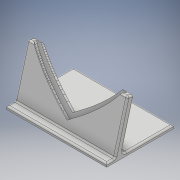
# Autodesk Inventor part: Supporto4
Saved by Autodesk Inventor 2018 (Build 220112000, 112)
## iProperties
Created: 2020-01-19
Part Number: Supporto4
Material: Generic
Document SubType Name: Modeling
Designer: Lorenzo Spadaro
Density: 1 g/cm^3
Appearance: Default
Author: Lorenzo Spadaro
Autodesk Inventor part; units mm, degrees
ref_plane "YZ Plane" through (0, 0, 0) normal (1, 0, 0) x (0, 1, 0)
ref_plane "XZ Plane" through (0, 0, 0) normal (0, 1, 0) x (-1, 0, 0)
ref_plane "XY Plane" through (0, 0, 0) normal (0, 0, 1) x (1, 0, 0)
sketch "Sketch1" plane through (0, 0, 0) normal (0, 0, 1) x (1, 0, 0)
  line L0 (-30, -20) -> (30, -20)
  line L1 (30, -20) -> (30, 20)
  line L2 (30, 20) -> (-30, 20)
  line L3 (-30, 20) -> (-30, -20)
  line L4 (-30, -20) -> (30, 20) construction
  line L5 (30, -20) -> (-30, 20) construction
  point P0 (0, 0)
  dimension "d0" = 60
  dimension "d1" = 40
  constraints: 12 end point, 2 midpoint, 2 parallel, 1 horizontal, 1 perpendicular
  measures "d0" distance of L2.end L1.end
  measures "d1" distance of L1.end L0.end
extrude "Extrusion1" add sketch "Sketch1" along normal blind 3
sketch "Sketch2" plane through (-30, -20, 0) normal (-1, 0, 0) x (0, 0, 1)
  line L0 (0, 0) -> (0, 40) projected
  line L1 (3, 40) -> (0, 40)
  line L2 (0, 40) -> (0, 0)
  line L3 (0, 0) -> (3, 0)
  line L4 (0, 40) -> (0, 20)
  line L5 (3, 40) -> (3, 5)
  line L6 (3, 5) -> (0, 5)
  line L7 (3, 0) -> (3, 40) projected
  line L8 (3, 5) -> (3, 0)
  line L9 (3, 5) -> (3, 9.4)
  line L10 (3, 9.4) -> (6, 9.4) construction
  line L11 (6.3002, 5.8843) -> (3, 5)
  line L12 (6.3002, 5.8843) -> (5.3582, 9.4)
  line L13 (6.3002, 5.8843) -> (9.9399, 5.8843) construction
  line L14 (5.3582, 9.4) -> (3, 9.4)
  dimension "d5" = 35
  dimension "d19" = 105
  dimension "d26" = 4.4
  dimension "d27" = 105
  constraints: 26 end point, 3 collinear, 3 horizontal, 3 point on line, 2 perpendicular, 1 equal length, 1 vertical
  measures "d5" distance of L1.start L5.end
  measures "d19" angle of L13 L12
  measures "d26" distance from line of L5.end L10
  measures "d27" angle of L7 L11
extrude "Extrusion2" add sketch "Sketch2" against normal blind 60 contours L5 L14 L12 L11
sketch "Sketch3" plane through (-30, -15, 3) normal (0, -0.9659258, 0.258819) x (1, 0, 0)
  line L0 (0, 3.4166) -> (60, 3.4166) projected
  line L1 (12.5923, 64.3215) -> (12.9587, 64.3506)
  line L2 (12.9587, 64.3506) -> (15.1774, 64.4331)
  line L3 (15.1774, 64.4331) -> (16.662, 64.3832)
  line L4 (16.662, 64.3832) -> (17.7697, 64.28)
  line L5 (17.7697, 64.28) -> (18.867, 64.1133)
  line L6 (18.867, 64.1133) -> (19.5902, 63.9637)
  line L7 (19.5902, 63.9637) -> (20.305, 63.7812)
  line L8 (20.305, 63.7812) -> (21.0099, 63.5638)
  line L9 (21.0099, 63.5638) -> (21.7034, 63.3097)
  line L10 (21.7034, 63.3097) -> (22.3839, 63.0169)
  line L11 (22.3839, 63.0169) -> (23.0499, 62.6836)
  line L12 (23.0499, 62.6836) -> (23.3315, 62.5336)
  line L13 (23.3315, 62.5336) -> (24.1498, 62.047)
  line L14 (24.1498, 62.047) -> (25.1851, 61.3212)
  line L15 (25.1851, 61.3212) -> (26.4008, 60.3111)
  line L16 (26.4008, 60.3111) -> (29.8855, 56.6294)
  line L17 (29.8855, 56.6294) -> (33.7036, 60.6652)
  line L18 (33.7036, 60.6652) -> (35.0763, 61.7545)
  line L19 (35.0763, 61.7545) -> (36.0566, 62.399)
  line L20 (36.0566, 62.399) -> (36.399, 62.6015)
  line L21 (36.399, 62.6015) -> (36.7462, 62.7923)
  line L22 (36.7462, 62.7923) -> (37.0981, 62.9719)
  line L23 (37.0981, 62.9719) -> (37.4543, 63.1403)
  line L24 (37.4543, 63.1403) -> (37.8145, 63.2978)
  line L25 (37.8145, 63.2978) -> (38.5466, 63.5813)
  line L26 (38.5466, 63.5813) -> (39.2924, 63.8242)
  line L27 (39.2924, 63.8242) -> (40.05, 64.0289)
  line L28 (40.05, 64.0289) -> (40.8179, 64.1969)
  line L29 (40.8179, 64.1969) -> (41.5938, 64.3304)
  line L30 (41.5938, 64.3304) -> (42.3761, 64.4315)
  line L31 (42.3761, 64.4315) -> (43.5574, 64.5263)
  line L32 (43.5574, 64.5263) -> (45.1374, 64.5574)
  line L33 (45.1374, 64.5574) -> (47.0997, 64.4654)
  line L34 (47.0997, 64.4654) -> (47.4823, 64.4315)
  line L35 (47.4823, 64.4315) -> (47.8629, 64.3861)
  line L36 (47.8629, 64.3861) -> (48.2415, 64.3295)
  line L37 (48.2415, 64.3295) -> (48.9917, 64.1836)
  line L38 (48.9917, 64.1836) -> (49.7314, 63.9952)
  line L39 (49.7314, 63.9952) -> (50.4592, 63.7661)
  line L40 (50.4592, 63.7661) -> (51.1737, 63.4979)
  line L41 (51.1737, 63.4979) -> (51.8735, 63.1921)
  line L42 (51.8735, 63.1921) -> (52.5571, 62.8503)
  line L43 (52.5571, 62.8503) -> (53.2231, 62.4741)
  line L44 (53.2231, 62.4741) -> (53.8701, 62.0653)
  line L45 (53.8701, 62.0653) -> (54.4966, 61.6253)
  line L46 (54.4966, 61.6253) -> (55.1012, 61.1557)
  line L47 (55.1012, 61.1557) -> (55.6826, 60.6582)
  line L48 (55.6826, 60.6582) -> (56.2392, 60.1345)
  line L49 (56.2392, 60.1345) -> (56.7697, 59.586)
  line L50 (56.7697, 59.586) -> (57.0867, 59.24)
  line L51 (57.0867, 59.24) -> (57.3931, 58.8859)
  line L52 (57.3931, 58.8859) -> (57.6888, 58.5239)
  line L53 (57.6888, 58.5239) -> (57.9739, 58.1544)
  line L54 (57.9739, 58.1544) -> (58.2485, 57.7777)
  line L55 (58.2485, 57.7777) -> (58.5128, 57.3941)
  line L56 (58.5128, 57.3941) -> (58.7666, 57.0037)
  line L57 (58.7666, 57.0037) -> (59.0103, 56.6072)
  line L58 (59.0103, 56.6072) -> (59.2438, 56.2044)
  line L59 (59.2438, 56.2044) -> (59.4672, 55.796)
  line L60 (59.4672, 55.796) -> (59.6807, 55.3819)
  line L61 (59.6807, 55.3819) -> (60.078, 54.5388)
  line L62 (60.078, 54.5388) -> (60.4362, 53.6772)
  line L63 (60.4362, 53.6772) -> (60.7561, 52.7996)
  line L64 (60.7561, 52.7996) -> (61.0385, 51.9084)
  line L65 (61.0385, 51.9084) -> (61.2838, 51.0058)
  line L66 (61.2838, 51.0058) -> (61.4928, 50.0942)
  line L67 (61.4928, 50.0942) -> (61.6662, 49.176)
  line L68 (61.6662, 49.176) -> (61.8045, 48.2534)
  line L69 (61.8045, 48.2534) -> (61.9085, 47.329)
  line L70 (61.9085, 47.329) -> (61.9254, 43.2771)
  line L71 (61.9254, 43.2771) -> (61.8677, 42.6923)
  line L72 (61.8677, 42.6923) -> (61.7957, 42.1069)
  line L73 (61.7957, 42.1069) -> (61.7102, 41.5244)
  line L74 (61.7102, 41.5244) -> (61.6114, 40.9447)
  line L75 (61.6114, 40.9447) -> (61.4997, 40.3679)
  line L76 (61.4997, 40.3679) -> (61.3754, 39.7942)
  line L77 (61.3754, 39.7942) -> (61.2388, 39.2235)
  line L78 (61.2388, 39.2235) -> (61.0903, 38.656)
  line L79 (61.0903, 38.656) -> (60.9299, 38.0918)
  line L80 (60.9299, 38.0918) -> (60.7584, 37.5308)
  line L81 (60.7584, 37.5308) -> (60.5757, 36.9731)
  line L82 (60.5757, 36.9731) -> (60.1784, 35.8681)
  line L83 (60.1784, 35.8681) -> (59.7408, 34.7775)
  line L84 (59.7408, 34.7775) -> (59.2652, 33.7017)
  line L85 (59.2652, 33.7017) -> (58.7541, 32.6411)
  line L86 (58.7541, 32.6411) -> (58.2101, 31.5965)
  line L87 (58.2101, 31.5965) -> (57.6357, 30.5684)
  line L88 (57.6357, 30.5684) -> (56.7225, 29.0583)
  line L89 (56.7225, 29.0583) -> (55.7548, 27.5883)
  line L90 (55.7548, 27.5883) -> (55.2622, 26.8873)
  line L91 (55.2622, 26.8873) -> (54.7597, 26.1941)
  line L92 (54.7597, 26.1941) -> (54.2477, 25.5087)
  line L93 (54.2477, 25.5087) -> (53.7265, 24.8308)
  line L94 (53.7265, 24.8308) -> (53.1963, 24.1603)
  line L95 (53.1963, 24.1603) -> (52.1103, 22.8408)
  line L96 (52.1103, 22.8408) -> (50.9918, 21.549)
  line L97 (50.9918, 21.549) -> (49.8431, 20.2836)
  line L98 (49.8431, 20.2836) -> (48.6664, 19.0434)
  line L99 (48.6664, 19.0434) -> (47.4641, 17.827)
  line L100 (47.4641, 17.827) -> (45.6174, 16.0446)
  line L101 (45.6174, 16.0446) -> (43.7254, 14.3087)
  line L102 (43.7254, 14.3087) -> (40.4923, 11.5077)
  line L103 (40.4923, 11.5077) -> (38.5167, 9.8753)
  line L104 (38.5167, 9.8753) -> (30.1085, 3.5424)
  line L105 (30.1085, 3.5424) -> (25.6132, 6.7843)
  line L106 (25.6132, 6.7843) -> (22.9564, 8.7926)
  line L107 (22.9564, 8.7926) -> (21.2085, 10.1624)
  line L108 (21.2085, 10.1624) -> (19.4827, 11.5593)
  line L109 (19.4827, 11.5593) -> (17.7822, 12.9857)
  line L110 (17.7822, 12.9857) -> (16.1101, 14.4435)
  line L111 (16.1101, 14.4435) -> (15.2856, 15.185)
  line L112 (15.2856, 15.185) -> (14.4694, 15.9352)
  line L113 (14.4694, 15.9352) -> (13.6619, 16.6943)
  line L114 (13.6619, 16.6943) -> (12.8633, 17.4626)
  line L115 (12.8633, 17.4626) -> (12.0742, 18.2405)
  line L116 (12.0742, 18.2405) -> (11.2948, 19.0283)
  line L117 (11.2948, 19.0283) -> (10.5256, 19.8261)
  line L118 (10.5256, 19.8261) -> (9.767, 20.6341)
  line L119 (9.767, 20.6341) -> (9.0194, 21.4528)
  line L120 (9.0194, 21.4528) -> (8.2831, 22.2824)
  line L121 (8.2831, 22.2824) -> (7.5585, 23.1231)
  line L122 (7.5585, 23.1231) -> (6.846, 23.9752)
  line L123 (6.846, 23.9752) -> (6.1461, 24.8391)
  line L124 (6.1461, 24.8391) -> (5.2953, 25.9462)
  line L125 (5.2953, 25.9462) -> (4.4707, 27.0787)
  line L126 (4.4707, 27.0787) -> (3.6761, 28.2357)
  line L127 (3.6761, 28.2357) -> (2.9153, 29.4166)
  line L128 (2.9153, 29.4166) -> (2.5487, 30.016)
  line L129 (2.5487, 30.016) -> (2.1921, 30.6211)
  line L130 (2.1921, 30.6211) -> (1.8457, 31.232)
  line L131 (1.8457, 31.232) -> (1.5103, 31.8485)
  line L132 (1.5103, 31.8485) -> (1.1861, 32.4705)
  line L133 (1.1861, 32.4705) -> (0.8737, 33.0981)
  line L134 (0.8737, 33.0981) -> (0.5736, 33.7312)
  line L135 (0.5736, 33.7312) -> (0.2862, 34.3696)
  line L136 (0.2862, 34.3696) -> (0.0121, 35.0132)
  line L137 (0.0121, 35.0132) -> (-0.2484, 35.6622)
  line L138 (-0.2484, 35.6622) -> (-0.4948, 36.3163)
  line L139 (-0.4948, 36.3163) -> (-0.7264, 36.9755)
  line L140 (-0.7264, 36.9755) -> (-0.943, 37.6397)
  line L141 (-0.943, 37.6397) -> (-1.144, 38.3089)
  line L142 (-1.144, 38.3089) -> (-1.3288, 38.9829)
  line L143 (-1.3288, 38.9829) -> (-1.4972, 39.6617)
  line L144 (-1.4972, 39.6617) -> (-1.6485, 40.3454)
  line L145 (-1.6485, 40.3454) -> (-1.7824, 41.0337)
  line L146 (-1.7824, 41.0337) -> (-1.8982, 41.7266)
  line L147 (-1.8982, 41.7266) -> (-1.9957, 42.424)
  line L148 (-1.9957, 42.424) -> (-2.0741, 43.1259)
  line L149 (-2.0741, 43.1259) -> (-2.0895, 46.8191)
  line L150 (-2.0895, 46.8191) -> (-1.9617, 48.0477)
  line L151 (-1.9617, 48.0477) -> (-1.776, 49.2715)
  line L152 (-1.776, 49.2715) -> (-1.5304, 50.4854)
  line L153 (-1.5304, 50.4854) -> (-1.2225, 51.6845)
  line L154 (-1.2225, 51.6845) -> (-0.8502, 52.8641)
  line L155 (-0.8502, 52.8641) -> (-0.5652, 53.6371)
  line L156 (-0.5652, 53.6371) -> (-0.2499, 54.3977)
  line L157 (-0.2499, 54.3977) -> (0.0962, 55.1443)
  line L158 (0.0962, 55.1443) -> (0.474, 55.8758)
  line L159 (0.474, 55.8758) -> (0.8839, 56.5905)
  line L160 (0.8839, 56.5905) -> (1.3267, 57.2868)
  line L161 (1.3267, 57.2868) -> (1.803, 57.9635)
  line L162 (1.803, 57.9635) -> (2.0705, 58.3169)
  line L163 (2.0705, 58.3169) -> (2.3475, 58.6637)
  line L164 (2.3475, 58.6637) -> (2.634, 59.0035)
  line L165 (2.634, 59.0035) -> (2.9297, 59.336)
  line L166 (2.9297, 59.336) -> (3.2344, 59.661)
  line L167 (3.2344, 59.661) -> (3.5476, 59.9781)
  line L168 (3.5476, 59.9781) -> (3.8693, 60.2869)
  line L169 (3.8693, 60.2869) -> (4.1992, 60.5872)
  line L170 (4.1992, 60.5872) -> (4.5371, 60.8785)
  line L171 (4.5371, 60.8785) -> (4.8827, 61.1605)
  line L172 (4.8827, 61.1605) -> (5.2358, 61.433)
  line L173 (5.2358, 61.433) -> (5.596, 61.6955)
  line L174 (5.596, 61.6955) -> (5.9633, 61.9478)
  line L175 (5.9633, 61.9478) -> (6.3373, 62.1896)
  line L176 (6.3373, 62.1896) -> (6.7178, 62.4204)
  line L177 (6.7178, 62.4204) -> (7.1046, 62.64)
  line L178 (7.1046, 62.64) -> (7.4974, 62.8481)
  line L179 (7.4974, 62.8481) -> (7.896, 63.0442)
  line L180 (7.896, 63.0442) -> (8.3001, 63.2281)
  line L181 (8.3001, 63.2281) -> (8.7095, 63.3995)
  line L182 (8.7095, 63.3995) -> (9.1239, 63.5579)
  line L183 (9.1239, 63.5579) -> (9.5432, 63.7031)
  line L184 (9.5432, 63.7031) -> (9.967, 63.8347)
  line L185 (9.967, 63.8347) -> (10.3952, 63.9525)
  line L186 (10.3952, 63.9525) -> (10.8274, 64.0561)
  line L187 (10.8274, 64.0561) -> (11.2635, 64.1451)
  line L188 (11.2635, 64.1451) -> (11.7031, 64.2192)
  line L189 (11.7031, 64.2192) -> (12.1462, 64.2781)
  line L190 (12.1462, 64.2781) -> (12.5923, 64.3215)
  line L191 (0, 0) -> (0, 3.4166) projected
  line L192 (0, 3.4166) -> (0, 29.4166)
  line L193 (0, 29.4166) -> (2.9153, 29.4166)
  line L194 (60, 3.4166) -> (60, 0) projected
  line L195 (60, 3.4166) -> (60, 29.4166)
  line L196 (60, 29.4166) -> (56.9392, 29.4166)
  point P0 (30, 0.9845)
  dimension "d15" = 26
  dimension "d16" = 26
  constraints: 388 end point, 4 perpendicular, 2 point on line, 1 horizontal, 1 parallel, 1 vertical
  measures "d15" distance of L0.start L192.end
  measures "d16" distance of L0.end L195.end
extrude "Extrusion3" add sketch "Sketch3" against normal blind 2.6 contours L192 L193 L127 L126 L125 L124 L123 L122 L121 L120 L119 L118 L117 L116 L115 L114 L113 L112 L111 L110 L109 L108 L107 L106 L105 L104 L103 L102 L101 L100 L99 L98 L97 L96 L95 L94 L93 L92 L91 L90 L89 L88 L196 L195 L0
sketch "Sketch4" plane through (26.9392, -7.3864, 31.4143) normal (0, 0.258819, 0.9659258) x (1, 0, 0)
  line L0 (3.0608, 2.6) -> (3.0608, 2.6) projected
  line L1 (-56.9392, 2.6) -> (-56.9392, 2.6) projected
  line L2 (-56.9392, 2.6) -> (3.0608, 2.6)
  line L3 (-56.9392, 5.4078) -> (3.0608, 5.4078) projected
  line L4 (-56.9392, 2.6) -> (-56.9392, 4.1)
  line L5 (-56.9392, 34.5839) -> (-56.9392, -4.0532) projected
  line L6 (-56.9392, 4.1) -> (3.0608, 4.1)
  line L7 (3.0608, 4.1) -> (3.0608, 2.6)
  line L8 (3.0608, -4.0532) -> (3.0608, 34.5839) projected
  point P0 (-26.9392, 15.2653)
  point P1 (-56.9392, 4.2501)
  point P2 (3.0608, 4.2501)
  dimension "d23" = 1.5
  constraints: 8 end point, 1 collinear, 1 perpendicular, 1 point on line
  measures "d23" distance of L1.start L4.end
extrude "Extrusion5" add sketch "Sketch4" against normal blind 28 contours L4 L6 L7 L2
sketch "Sketch6" plane through (-27.0847, -4.875, 30.7413) normal (0, -0.9659258, 0.258819) x (1, 0, 0)
  line L0 (37.577, -17.9089) -> (40.8101, -15.108) projected
  line L1 (40.8101, -15.108) -> (42.702, -13.372) projected
  line L2 (42.702, -13.372) -> (44.5488, -11.5896) projected
  line L3 (44.5488, -11.5896) -> (45.7511, -10.3732) projected
  line L4 (45.7511, -10.3732) -> (46.9277, -9.133) projected
  line L5 (46.9277, -9.133) -> (48.0764, -7.8676) projected
  line L6 (48.0764, -7.8676) -> (49.1949, -6.5758) projected
  line L7 (49.1949, -6.5758) -> (50.2809, -5.2563) projected
  line L8 (50.2809, -5.2563) -> (50.8111, -4.5858) projected
  line L9 (50.8111, -4.5858) -> (51.3324, -3.9079) projected
  line L10 (51.3324, -3.9079) -> (51.8443, -3.2225) projected
  line L11 (51.8443, -3.2225) -> (52.3468, -2.5294) projected
  line L12 (52.3468, -2.5294) -> (52.8395, -1.8283) projected
  line L13 (52.8395, -1.8283) -> (53.8072, -0.3583) projected
  line L14 (53.8072, -0.3583) -> (54.0239, 0) projected
  line L15 (2.3799, 0.5296) -> (3.2308, -0.5775)
  line L16 (3.2308, -0.5775) -> (3.9307, -1.4414)
  line L17 (3.9307, -1.4414) -> (4.6432, -2.2935)
  line L18 (4.6432, -2.2935) -> (5.3678, -3.1342)
  line L19 (5.3678, -3.1342) -> (6.1041, -3.9638)
  line L20 (6.1041, -3.9638) -> (6.8517, -4.7825)
  line L21 (6.8517, -4.7825) -> (7.6103, -5.5905)
  line L22 (7.6103, -5.5905) -> (8.3794, -6.3883)
  line L23 (8.3794, -6.3883) -> (9.1588, -7.1761)
  line L24 (9.1588, -7.1761) -> (9.948, -7.954)
  line L25 (9.948, -7.954) -> (10.7465, -8.7223)
  line L26 (10.7465, -8.7223) -> (11.5541, -9.4815)
  line L27 (11.5541, -9.4815) -> (12.3703, -10.2317)
  line L28 (12.3703, -10.2317) -> (13.1948, -10.9731)
  line L29 (13.1948, -10.9731) -> (14.8669, -12.4309)
  line L30 (14.8669, -12.4309) -> (16.5674, -13.8573)
  line L31 (16.5674, -13.8573) -> (18.2931, -15.2542)
  line L32 (18.2931, -15.2542) -> (20.0411, -16.624)
  line L33 (20.0411, -16.624) -> (22.6979, -18.6323)
  line L34 (22.6979, -18.6323) -> (27.1932, -21.8742)
  line L35 (27.1932, -21.8742) -> (35.6014, -15.5413)
  line L36 (35.6014, -15.5413) -> (37.577, -13.9089)
  line L37 (37.577, -13.9089) -> (40.8101, -11.108)
  line L38 (40.8101, -11.108) -> (42.702, -9.372)
  line L39 (42.702, -9.372) -> (44.5488, -7.5896)
  line L40 (44.5488, -7.5896) -> (45.7511, -6.3732)
  line L41 (45.7511, -6.3732) -> (46.9277, -5.133)
  line L42 (46.9277, -5.133) -> (48.0764, -3.8676)
  line L43 (48.0764, -3.8676) -> (49.1949, -2.5758)
  line L44 (49.1949, -2.5758) -> (50.2809, -1.2563)
  line L45 (50.2809, -1.2563) -> (50.8111, -0.5858)
  line L46 (50.8111, -0.5858) -> (51.3324, 0.0921)
  line L47 (27.1932, -25.8742) -> (35.6014, -19.5413) projected
  line L48 (27.1932, -21.8742) -> (27.1932, -25.8742)
  line L49 (0, 0) -> (54.0239, 0) projected
  line L50 (51.2616, 0) -> (2.787, 0)
  point P0 (27.0847, -28.4321)
  constraints: 68 end point, 4 point on line, 1 vertical
extrude "Extrusion7" cut sketch "Sketch6" against normal blind 2
sketch "Sketch7" plane through (-30, -15, 3) normal (0, -0.9659258, 0.258819) x (1, 0, 0)
  line L0 (47.4641, 17.827) -> (45.6174, 16.0446) projected
  line L1 (45.6174, 16.0446) -> (47.4641, 17.827) projected
  line L2 (60, 29.4166) -> (56.9392, 29.4166) projected
  line L3 (0, 0) -> (0, 29.4166) projected
  line L4 (60, 0) -> (0, 0) projected
  line L5 (60, 0) -> (60, 29.4166) projected
  line L6 (60, 29.4166) -> (56.9392, 29.4166) projected
  line L7 (56.9392, 29.4166) -> (56.7225, 29.0583) projected
  line L8 (56.7225, 29.0583) -> (55.7548, 27.5883) projected
  line L9 (55.7548, 27.5883) -> (55.2622, 26.8873) projected
  line L10 (55.2622, 26.8873) -> (54.7597, 26.1941) projected
  line L11 (54.7597, 26.1941) -> (54.2477, 25.5087) projected
  line L12 (54.2477, 25.5087) -> (53.7265, 24.8308) projected
  line L13 (53.7265, 24.8308) -> (53.1963, 24.1603) projected
  line L14 (53.1963, 24.1603) -> (52.1103, 22.8408) projected
  line L15 (52.1103, 22.8408) -> (50.9918, 21.549) projected
  line L16 (50.9918, 21.549) -> (49.8431, 20.2836) projected
  line L17 (49.8431, 20.2836) -> (48.6664, 19.0434) projected
  line L18 (48.6664, 19.0434) -> (47.4641, 17.827) projected
  line L19 (47.4641, 17.827) -> (45.6174, 16.0446) projected
  line L20 (45.6174, 16.0446) -> (43.7254, 14.3087) projected
  line L21 (43.7254, 14.3087) -> (40.4923, 11.5077) projected
  line L22 (40.4923, 11.5077) -> (38.5167, 9.8753) projected
  line L23 (38.5167, 9.8753) -> (30.1085, 3.5424) projected
  line L24 (30.1085, 3.5424) -> (25.6132, 6.7843) projected
  line L25 (25.6132, 6.7843) -> (22.9564, 8.7926) projected
  line L26 (22.9564, 8.7926) -> (21.2085, 10.1624) projected
  line L27 (21.2085, 10.1624) -> (19.4827, 11.5593) projected
  line L28 (19.4827, 11.5593) -> (17.7822, 12.9857) projected
  line L29 (17.7822, 12.9857) -> (16.1101, 14.4435) projected
  line L30 (16.1101, 14.4435) -> (15.2856, 15.185) projected
  line L31 (15.2856, 15.185) -> (14.4694, 15.9352) projected
  line L32 (14.4694, 15.9352) -> (13.6619, 16.6943) projected
  line L33 (13.6619, 16.6943) -> (12.8633, 17.4626) projected
  line L34 (12.8633, 17.4626) -> (12.0742, 18.2405) projected
  line L35 (12.0742, 18.2405) -> (11.2948, 19.0283) projected
  line L36 (11.2948, 19.0283) -> (10.5256, 19.8261) projected
  line L37 (10.5256, 19.8261) -> (9.767, 20.6341) projected
  line L38 (9.767, 20.6341) -> (9.0194, 21.4528) projected
  line L39 (9.0194, 21.4528) -> (8.2831, 22.2824) projected
  line L40 (8.2831, 22.2824) -> (7.5585, 23.1231) projected
  line L41 (7.5585, 23.1231) -> (6.846, 23.9752) projected
  line L42 (6.846, 23.9752) -> (6.1461, 24.8391) projected
  line L43 (6.1461, 24.8391) -> (5.2953, 25.9462) projected
  line L44 (5.2953, 25.9462) -> (4.4707, 27.0787) projected
  line L45 (4.4707, 27.0787) -> (3.6761, 28.2357) projected
  line L46 (3.6761, 28.2357) -> (2.9153, 29.4166) projected
  line L47 (2.9153, 29.4166) -> (0, 29.4166) projected
  line L48 (30.1085, 3.5424) -> (25.6132, 6.7843) projected
  line L49 (30.1085, 3.5424) -> (30.1085, 4.5424)
  line L50 (47.4641, 18.6844) -> (45.6174, 16.902)
  line L51 (45.6174, 16.902) -> (47.4641, 18.6844)
  line L52 (56.9392, 30.4166) -> (56.7225, 30.0583)
  line L53 (56.7225, 30.0583) -> (55.7548, 28.5883)
  line L54 (55.7548, 28.5883) -> (55.2622, 27.8873)
  line L55 (55.2622, 27.8873) -> (54.7597, 27.1941)
  line L56 (54.7597, 27.1941) -> (54.2477, 26.5087)
  line L57 (54.2477, 26.5087) -> (53.7265, 25.8308)
  line L58 (53.7265, 25.8308) -> (53.1963, 25.1603)
  line L59 (53.1963, 25.1603) -> (52.1103, 23.8408)
  line L60 (52.1103, 23.8408) -> (50.9918, 22.549)
  line L61 (50.9918, 22.549) -> (49.8431, 21.2836)
  line L62 (49.8431, 21.2836) -> (48.6664, 20.0434)
  line L63 (48.6664, 20.0434) -> (47.4641, 18.827)
  line L64 (47.4641, 18.827) -> (45.6174, 17.0446)
  line L65 (45.6174, 17.0446) -> (43.7254, 15.3087)
  line L66 (43.7254, 15.3087) -> (40.4923, 12.5077)
  line L67 (40.4923, 12.5077) -> (38.5167, 10.8753)
  line L68 (38.5167, 10.8753) -> (30.1085, 4.5424)
  line L69 (30.1085, 4.5424) -> (25.6132, 7.7843)
  line L70 (25.6132, 7.7843) -> (22.9564, 9.7926)
  line L71 (22.9564, 9.7926) -> (21.2085, 11.1624)
  line L72 (21.2085, 11.1624) -> (19.4827, 12.5593)
  line L73 (19.4827, 12.5593) -> (17.7822, 13.9857)
  line L74 (17.7822, 13.9857) -> (16.1101, 15.4435)
  line L75 (16.1101, 15.4435) -> (15.2856, 16.185)
  line L76 (15.2856, 16.185) -> (14.4694, 16.9352)
  line L77 (14.4694, 16.9352) -> (13.6619, 17.6943)
  line L78 (13.6619, 17.6943) -> (12.8633, 18.4626)
  line L79 (12.8633, 18.4626) -> (12.0742, 19.2405)
  line L80 (12.0742, 19.2405) -> (11.2948, 20.0283)
  line L81 (11.2948, 20.0283) -> (10.5256, 20.8261)
  line L82 (10.5256, 20.8261) -> (9.767, 21.6341)
  line L83 (9.767, 21.6341) -> (9.0194, 22.4528)
  line L84 (9.0194, 22.4528) -> (8.2831, 23.2824)
  line L85 (8.2831, 23.2824) -> (7.5585, 24.1231)
  line L86 (7.5585, 24.1231) -> (6.846, 24.9752)
  line L87 (6.846, 24.9752) -> (6.1461, 25.8391)
  line L88 (6.1461, 25.8391) -> (5.2953, 26.9462)
  line L89 (5.2953, 26.9462) -> (4.4707, 28.0787)
  line L90 (4.4707, 28.0787) -> (3.6761, 29.2357)
  line L91 (3.6761, 29.2357) -> (2.9153, 30.4166)
  line L92 (3.6761, 28.2357) -> (2.9153, 29.4166) projected
  line L93 (2.9153, 29.4166) -> (3.5595, 29.4166)
  line L94 (56.9392, 29.4166) -> (56.3001, 29.4166)
  point P0 (30, 0.9845)
  point P1 (56.9392, 30.274)
  dimension "d44" = 1
  constraints: 90 end point, 6 point on line, 1 vertical
  measures "d44" distance of L23.end L49.end
extrude "Extrusion8" add sketch "Sketch7" against normal blind 0.5 contours L0 L20 L21 L22 L23 L49 L68 L67 L66 L65 L64 L63 L62 L61 L60 L59 L58 L57 L56 L55 L54 L53 L94 L7 L8 L9 L10 L11 L12 L13 L14 L15 L16 L17 L18 | L24 L25 L26 L27 L28 L29 L30 L31 L32 L33 L34 L35 L36 L37 L38 L39 L40 L41 L42 L43 L44 L45 L46 L93 L91 L90 L89 L88 L87 L86 L85 L84 L83 L82 L81 L80 L79 L78 L77 L76 L75 L74 L73 L72 L71 L70 L69 L49
fillet "Fillet4" radius 2 2 edges at (0, -10.6, 3.5798) (0, -10.6, 3)
sketch "Sketch8" plane through (0, 0, 3) normal (0, 0, 1) x (1, 0, 0)
  line L0 (24, -5.1489) -> (21, -5.1489)
  line L1 (21, -5.1489) -> (21, -7.1489)
  line L2 (21, -7.1489) -> (24, -7.1489)
  line L3 (24, -7.1489) -> (24, -5.1489)
  line L4 (-21, -5.1489) -> (-24, -5.1489)
  line L5 (-24, -5.1489) -> (-24, -7.1475)
  line L6 (-24, -7.1475) -> (-21, -7.1475)
  line L7 (-21, -7.1475) -> (-21, -5.1489)
  line L8 (-24, -5.1489) -> (-29, -5.1489)
  line L9 (29, -5.1489) -> (24, -5.1489)
  line L10 (29, -4.8774) -> (29, 20)
  line L11 (30, 20) -> (-30, 20) projected
  line L12 (-29, -5.1489) -> (-29, 20)
  line L13 (30, -8.1489) -> (30, 20) projected
  line L14 (29, -4.8774) -> (29, -5.1489)
  line L15 (29, -5.1489) -> (29, -8.1489)
  line L16 (-29, -5.1489) -> (-29, -8.1489)
  line L17 (-29, -8.1489) -> (-30, -8.1489)
  line L18 (-29, -8.1489) -> (29, -8.1489)
  line L19 (30, -8.1489) -> (-30, -8.1489) projected
  point P0 (0, 0)
  dimension "d51" = 3
  dimension "d52" = 2
  dimension "d53" = 3
  dimension "d54" = 42
  dimension "d55" = 3
  dimension "d56" = 5
  dimension "d62" = 27.1474
  dimension "d63" = 24.8774
  constraints: 34 end point, 9 perpendicular, 3 point on line, 3 vertical, 1 collinear, 1 horizontal, 1 parallel
  measures "d51" distance of L0.start L0.end
  measures "d52" distance of L0.end L1.end
  measures "d53" distance of L1.end L2.end
  measures "d54" distance of L0.end L4.start
  measures "d55" distance of L4.start L4.end
  measures "d56" distance of L4.end L8.end
  measures "d62" distance between parallel lines of L6 L11
  measures "d63" distance from line of L10.start L11
extrude "Extrusion9" add sketch "Sketch8" along normal up to next contours L3 L2 L1 L0 | L7 L6 L5 L4
fillet "Fillet7" radius 0.5 16 edges at (-21, -5.1489, 13.4618) (-21, -7.1475, 9.7325) (-24, -5.1489, 13.4618) (-24, -7.1475, 9.7325) (21, -5.1489, 13.4618) (21, -7.1489, 9.7297) (24, -5.1489, 13.4618) (24, -7.1489, 9.7297) (24, -6.1489, 3) (22.5, -7.1489, 3) (21, -6.1489, 3) (22.5, -5.1489, 3) (-24, -6.1482, 3) (-22.5, -5.1489, 3) (-21, -6.1482, 3) (-22.5, -7.1475, 3)
fillet "Fillet8" radius 1 19 edges at (-30, -9.7356, 3.7825) (-30, -6.7534, 17.9354) (-30, 5.9255, 3) (30, -9.7356, 3.7825) (30, 5.9255, 3) (30, -6.7534, 17.9354) (30, -11.1932, 17.2071) (30, -17.5, 3) (0, 20, 3) (27.0885, -3.4261, 30.3531) (30, -5.4063, 30.8837) (28.15, -7.3864, 31.4143) (-30, -5.4063, 30.8837) (-27.1489, -3.4261, 30.3531) (-28.2202, -7.3864, 31.4143) (0, -20, 3) (-30, -17.5, 3) (-30, -11.1932, 17.2071) (0, -15, 3)
sketch "Sketch10" plane through (0, 0, 0) normal (0, 0, -1) x (-1, 0, 0)
  line L0 (30, -20) -> (-30, -20) projected
  line L1 (30, 20.0775) -> (30, -20)
  line L2 (30, -20) -> (-30, -20)
  line L3 (-30, 20) -> (30, 20) projected
  line L4 (-30, -20) -> (-30, 20)
  line L5 (-30, 20) -> (30, 20)
  point P0 (0, 0)
  constraints: 8 end point, 4 perpendicular
extrude "Extrusion10" cut sketch "Sketch10" against normal blind 1
body "Solid1"
